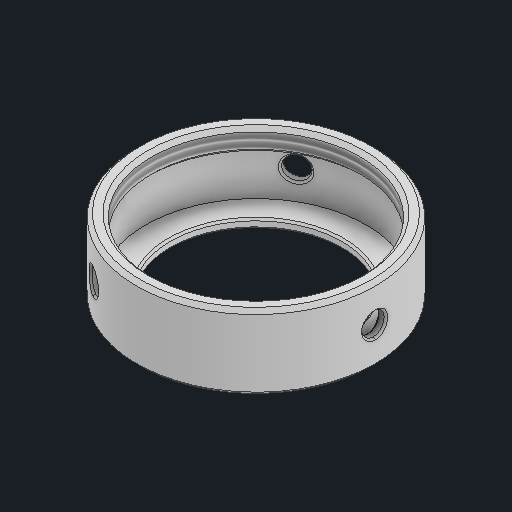
# Autodesk Inventor part: 017
Saved by Autodesk Inventor 2022 (Build 260153000, 153)
## iProperties
Created: 2021-11-15
Part Number: 017
Material: Generic
Document SubType Name: Modeling
Designer: vinicius.miguel
Density: 1 g/cm^3
Appearance: Default
Mass: 1.62672 g
Surface Area: 26.7009 cm^2
Volume: 1.62672 cm^3
Author: vinicius.miguel
Autodesk Inventor part; units mm, degrees
ref_plane "XZ Plane" through (0, 0, 0) normal (0, 1, 0) x (-1, 0, 0)
ref_plane "XY Plane" through (0, 0, 0) normal (0, 0, 1) x (1, 0, 0)
sketch "Sketch1" plane through (0, 0, 0) normal (0, 0, 1) x (1, 0, 0)
  line L0 (0, 0) -> (0, 7.8624)
  line L1 (11.5, 0) -> (11.5, 1.2)
  line L2 (11.5, 1.2) -> (14.8, 1.2)
  line L3 (14.8, 1.2) -> (14.8, 7)
  line L4 (14.8, 7) -> (14, 7)
  line L5 (14, 7) -> (14, 10)
  line L6 (14, 10) -> (16, 10)
  line L7 (16, 10) -> (16, 0.5)
  line L8 (15.5, 0) -> (11.5, 0)
  line L9 (16, 0.5) -> (15.5, 0)
  point P0 (16, 0)
  dimension "d0" = 23
  dimension "d1" = 1.2
  dimension "d2" = 1.2
  dimension "d3" = 2
  dimension "d4" = 32
  dimension "d5" = 3
  dimension "d6" = 10
  dimension "d8" = 0.5
  dimension "d9" = 0.5
  constraints: 20 end point, 7 perpendicular, 2 point on line, 2 vertical, 1 horizontal alignment
  measures "d0" diameter of L1 L0
  measures "d1" distance of L1.start L1.end
  measures "d2" distance between parallel lines of L7 L3
  measures "d3" distance between parallel lines of L7 L5
  measures "d4" diameter of L7 L0
  measures "d5" distance of L4.end L5.end
  measures "d6" distance from line of L6 L0.start
  measures "d8" distance of L7.end point (16, 0)
  measures "d9" distance of L8.start point (16, 0)
revolve "Revolution1" add sketch "Sketch1" angle 360 about axis through (0, 0, 0) along (0, 1, 0)
chamfer "Chamfer1" distance 0.5 angle 45 1 edges at (-16, 10, 0)
thread "Thread1" size "M28x1" class "6H" standard "ANSI Metric M Profile" full length
chamfer "Chamfer2" distance 0.25 angle 45 2 edges at (-11.5, 1.2, 0) (-11.5, 0, 0)
chamfer "Chamfer3" distance 0.5 angle 45 2 edges at (-14, 10, 0) (-14, 7, 0)
ref_plane "Work Plane1" through (16, 5.25, 0) normal (1, 0, 0) x (0, 1, 0)
sketch "Sketch2" plane through (16, 5.25, 0) normal (1, 0, 0) x (0, 1, 0)
  line L0 (4.25, 16) -> (-4.75, 16) projected
  point P0 (-5.25, 0)
  point P1 (-0.25, 0)
  point P2 (-0.25, 16)
  constraints: 1 horizontal alignment, 1 midpoint, 1 vertical alignment
hole "Hole1" at (16, 5, 0) direction (-1, 0, 0) diameter 3 depth 5
chamfer "Chamfer4" distance 0.25 angle 45 6 edges at (14.7567, 4.0149, -1.1312) (14.7238, 4.9998, 1.5) (14.7568, 5.9868, -1.1297) (15.96, 4.0149, -1.1312) (15.9601, 5.9867, -1.1297) (15.9295, 4.9998, 1.5)
pattern_circular "Circular Pattern1" count 3 over 360 about axis through (0, 5.25, 0) along (0, -1, 0) of "Hole1", "Chamfer4"
equation "\"d9\" = d8"
body "Solid1"
